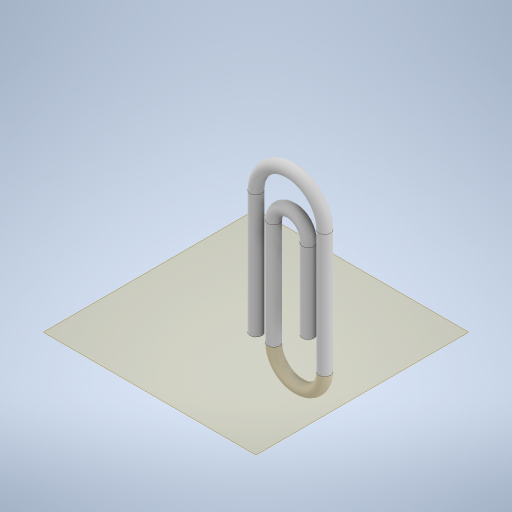
# Autodesk Inventor part: paperclip
Saved by Autodesk Inventor 2024 (Build 280153000, 153)
## iProperties
Created: 2023-10-05
Part Number: paperclip
Material: Generic
Document SubType Name: Modeling
Designer: Arshan
Density: 1 g/cm^3
Appearance: Default
Author: Arshan
Autodesk Inventor part; units mm, degrees
ref_plane "YZ Plane" through (0, 0, 0) normal (1, 0, 0) x (0, 1, 0)
ref_plane "XZ Plane" through (0, 0, 0) normal (0, 1, 0) x (-1, 0, 0)
ref_plane "XY Plane" through (0, 0, 0) normal (0, 0, 1) x (1, 0, 0)
sketch "Sketch1" plane through (0, 0, 0) normal (0, 0, 1) x (1, 0, 0)
  line L0 (4.6732, 5.2798) -> (4.6732, 18.0188)
  arc A0 (11.7729, 18.0188) -> (4.6732, 18.0188) centre (8.223, 18.0188) ccw
  line L1 (11.7729, 18.0188) -> (11.7729, 5.2798)
  arc A1 (6.5003, 5.2798) -> (11.7729, 5.2798) centre (9.1366, 5.2798) ccw
  line L2 (6.5003, 5.2798) -> (6.5003, 16.2299)
  arc A2 (10.0653, 15.9967) -> (6.5003, 16.2299) centre (8.2904, 16.2299) ccw
  line L3 (10.0653, 15.9967) -> (10.0653, 7.7471)
  point P0 (0, 0)
  constraints: 8 end point, 7 point on circle, 4 vertical, 3 centre point, 3 tangent
ref_plane "Work Plane1" through (4.6732, 5.2798, 0) normal (0, 1, 0) x (-1, 0, 0)
sketch "Sketch2" plane through (4.6732, 5.2798, 0) normal (0, 1, 0) x (-1, 0, 0)
  circle A0 centre (0, 0) radius 0.6158
  point P0 (4.6732, 0)
  constraints: 1 centre point
sweep "Sweep1" add profiles "Sketch2" path "Sketch1"
body "Solid1"
